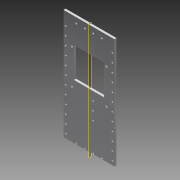
# Autodesk Inventor part: YagiTop
Saved by Autodesk Inventor 2014 (Build 180170000, 170)
## iProperties
Created: 2015-04-18
Part Number: YagiTop
Material: Generic
Document SubType Name: Modeling
Designer: Owner
Density: 1 g/cm^3
Appearance: Aluminum - Polished
Author: Owner
Autodesk Inventor part; units mm, degrees
ref_plane "YZ Plane" through (0, 0, 0) normal (1, 0, 0) x (0, 1, 0)
ref_plane "XZ Plane" through (0, 0, 0) normal (0, 1, 0) x (-1, 0, 0)
ref_plane "XY Plane" through (0, 0, 0) normal (0, 0, 1) x (1, 0, 0)
sketch "Sketch1" plane through (0, 0, 0) normal (0, 0, 1) x (1, 0, 0)
  line L0 (4.9626, 165.1) -> (81.1626, 165.1)
  line L1 (81.1626, 165.1) -> (81.1626, 0)
  line L2 (81.1626, 0) -> (4.9626, 0)
  line L3 (4.9626, 0) -> (4.9626, 165.1)
  point P0 (0, 0)
  dimension "d0" = 76.2
  dimension "d1" = 165.1
  constraints: 8 end point, 2 parallel, 1 horizontal, 1 perpendicular
  measures "d0" distance of L1.end L2.end
  measures "d1" distance of L0.end L1.end
extrude "Extrusion1" add sketch "Sketch1" along normal blind 3.175
sketch "Sketch2" plane through (0, 0, 3.175) normal (0, 0, 1) x (1, 0, 0)
  line L0 (81.1626, 165.1) -> (4.9626, 165.1) projected
  line L1 (81.1626, 0) -> (81.1626, 165.1) projected
  line L2 (20.5626, 127) -> (65.5626, 127)
  line L3 (65.5626, 127) -> (65.5626, 82)
  line L4 (65.5626, 82) -> (20.5626, 82)
  line L5 (20.5626, 82) -> (20.5626, 127)
  point P0 (0, 0)
  dimension "d4" = 45
  dimension "d5" = 45
  dimension "d6" = 15.6
  dimension "d7" = 38.1
  constraints: 8 end point, 2 parallel, 1 horizontal, 1 perpendicular
  measures "d4" distance of L2.start L2.end
  measures "d5" distance of L4.end L2.start
  measures "d6" distance between parallel lines of L1 L3
  measures "d7" distance between parallel lines of L0 L2
extrude "Extrusion2" cut sketch "Sketch2" against normal blind 3.175
sketch "Sketch3" plane through (0, 0, 0) normal (0, 0, -1) x (-1, 0, 0)
  point P0 (-69.0626, 78.5)
hole "Hole1" at (69.0626, 78.5, 0) direction (0, 0, 1) diameter 3.4544 depth 3.175
sketch "Sketch4" plane through (0, 0, 0) normal (0, 0, -1) x (-1, 0, 0)
  point P0 (-17.0626, 78.5)
hole "Hole3" at (17.0626, 78.5, 0) direction (0, 0, 1) diameter 3.4544 depth 3.175
sketch "Sketch5" plane through (0, 0, 0) normal (0, 0, -1) x (-1, 0, 0)
  point P0 (-69.0626, 130.5)
hole "Hole5" at (69.0626, 130.5, 0) direction (0, 0, 1) diameter 3.4544 depth 3.175
sketch "Sketch6" plane through (0, 0, 0) normal (0, 0, -1) x (-1, 0, 0)
  point P0 (-17.0626, 130.5)
hole "Hole7" at (17.0626, 130.5, 0) direction (0, 0, 1) diameter 3.4544 depth 3.175
sketch "Sketch7" plane through (0, 0, 3.175) normal (0, 0, 1) x (1, 0, 0)
  point P0 (49.4126, 75.65)
hole "Hole9" at (49.4126, 75.65, 3.175) direction (0, 0, -1) diameter 1.778 depth 3.175 countersink diameter 3.0226 countersink angle 82
pattern_linear "Rectangular Pattern1" count 3 spacing 12.7 along (0, -1, 0) of "Hole9"
sketch "Sketch8" plane through (0, 0, 3.175) normal (0, 0, 1) x (1, 0, 0)
  point P0 (24.0126, 3.175)
hole "Hole11" at (24.0126, 3.175, 3.175) direction (0, 0, -1) diameter 1.778 depth 3.175 countersink diameter 3.0226 countersink angle 82
sketch "Sketch9" plane through (0, 0, 3.175) normal (0, 0, 1) x (1, 0, 0)
  point P0 (8.1376, 12.7)
hole "Hole13" at (8.1376, 12.7, 3.175) direction (0, 0, -1) diameter 1.778 depth 3.175 countersink diameter 3.0226 countersink angle 100
pattern_linear "Rectangular Pattern3" count 12 spacing 12.7 along (0, 1, 0) of "Hole13"
ref_plane "Work Plane1" through (43.0626, 0, 0) normal (-1, 0, 0) x (0, 0, 1)
sketch "Sketch10" plane through (0, 0, 3.175) normal (0, 0, 1) x (1, 0, 0)
  point P0 (24.0126, 161.925)
hole "Hole15" at (24.0126, 161.925, 3.175) direction (0, 0, -1) diameter 1.778 depth 3.175 countersink diameter 3.0226 countersink angle 82
pattern_linear "Rectangular Pattern4" count 2 spacing 12.7 along (1, 0, 0) of "Hole15"
pattern_linear "Rectangular Pattern5" count 2 spacing 12.7 along (1, 0, 0) of "Hole11"
mirror "Mirror1" about plane through (43.0626, 0, 0) normal (-1, 0, 0) of "Hole11", "Hole13", "Rectangular Pattern3", "Hole15", "Rectangular Pattern4", "Rectangular Pattern5"
ref_plane "Work Plane2" through (43.0626, 0, 0) normal (-1, 0, 0) x (0, 0, 1)
body "Solid1"
